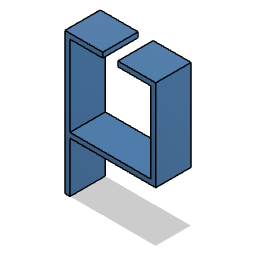
CryoKit_Clip_V2.4.7 (Autodesk Fusion 360 design; units mm, degrees)
Autodesk Fusion 360 part; units mm, degrees
sketch "Sketch1" plane through (0, 0, 0) normal (0, 0, 1) x (-1, 0, 0)
  line L0 (8, -8) -> (-8, -8)
  line L1 (-8, -8) -> (-8, 8)
  line L2 (-8, 8) -> (8, 8)
  line L3 (8, 8) -> (8, -8)
  line L4 (8, -8) -> (-8, 8) construction
  line L5 (-8, -8) -> (8, 8) construction
  line L6 (9, -9) -> (-9, -9)
  line L7 (-9, -9) -> (-9, 9)
  line L8 (-9, 9) -> (9, 9)
  line L9 (9, 9) -> (9, -9)
  line L10 (9, -9) -> (-9, 9) construction
  line L11 (-9, -9) -> (9, 9) construction
  line L12 (1.5, -9) -> (-1.5, -9)
  line L13 (-1.5, -9) -> (-1.5, -8)
  line L14 (-1.5, -8) -> (1.5, -8)
  line L15 (1.5, -8) -> (1.5, -9)
  line L16 (1.5, -9) -> (-1.5, -8) construction
  line L17 (-1.5, -9) -> (1.5, -8) construction
  line L18 (9, 9) -> (8, 9)
  line L19 (8, 9) -> (8, 19)
  line L20 (8, 19) -> (9, 19)
  line L21 (9, 19) -> (9, 9)
  point P0 (0, -8.5)
  dimension "d1" = 16
  dimension "d2" = 16
  dimension "d3" = 18
  dimension "d4" = 18
  dimension "d5" = 3
  dimension "d6" = 1
  dimension "d7" = 1
  dimension "d8" = 10
  constraint horizontal L0
  constraint perpendicular L0 L1
  constraint parallel L0 L2
  constraint parallel L1 L3
  constraint coincident L4 origin
  constraint coincident L5 origin
  constraint horizontal L6
  constraint perpendicular L6 L7
  constraint parallel L6 L8
  constraint parallel L7 L9
  constraint coincident L10 origin
  constraint coincident L11 origin
  constraint horizontal L12
  constraint perpendicular L12 L13
  constraint parallel L12 L14
  constraint parallel L13 L15
  constraint coincident L16 P0
  constraint coincident L17 P0
  constraint horizontal L18
  constraint vertical L19
  constraint horizontal L20
  constraint vertical L21
  measures "d1" distance of L1.end L2.end
  measures "d2" distance of L0.end L1.end
  measures "d3" distance of L7.end L8.end
  measures "d4" distance of L6.end L7.end
  measures "d5" distance of L13.end L14.end
  measures "d6" distance of L12.end L13.end
  measures "d7" distance of L8.end L18.end
  measures "d8" distance of L8.end L20.end
extrude "Extrude1" add sketch "Sketch1" along normal blind 7 contours L0 L1 L2 L3 L6 L7 L8 L9 L13 L15 L18 | L8 L18 L19 L20 L21
